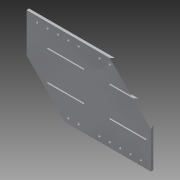
# Autodesk Inventor part: LiDAR Plate
Saved by Autodesk Inventor 2016 (Build 200138000, 138)
## iProperties
Created: 2016-04-02
Part Number: LiDAR Plate
Material: Aluminum 6061
Document SubType Name: Modeling
Designer: hwasserb
Density: 2.71 g/cm^3
Appearance: Aluminum - Flat
Author: hwasserb
Autodesk Inventor part; units mm, degrees
ref_plane "YZ Plane" through (0, 0, 0) normal (1, 0, 0) x (0, 1, 0)
ref_plane "XZ Plane" through (0, 0, 0) normal (0, 1, 0) x (-1, 0, 0)
ref_plane "XY Plane" through (0, 0, 0) normal (0, 0, 1) x (1, 0, 0)
sketch "Sketch1" plane through (0, 0, 0) normal (0, 1, 0) x (-1, 0, 0)
  line L0 (0, 0) -> (-304.8, 0)
  line L1 (-304.8, 0) -> (-304.8, 190.5)
  line L2 (-304.8, 190.5) -> (0, 190.5)
  line L3 (0, 190.5) -> (0, 0)
  dimension "d0" = 304.8
  dimension "d1" = 190.5
  constraints: 8 end point, 2 parallel, 1 horizontal, 1 perpendicular
  measures "d0" distance of L0.start L0.end
  measures "d1" distance of L2.end L0.start
extrude "Extrusion1" add sketch "Sketch1" along normal blind 6.35
sketch "Sketch2" plane through (0, 6.35, 0) normal (0, 1, 0) x (1, 0, 0)
  line L0 (304.8, 0) -> (0, 0) projected
  line L1 (0, 0) -> (0, -190.5) projected
  line L2 (0, -190.5) -> (304.8, -190.5) projected
  line L3 (304.8, -190.5) -> (304.8, 0) projected
  point P0 (25.4, -12.7)
  point P1 (50.8, -12.7)
  point P2 (76.2, -12.7)
  point P3 (101.6, -12.7)
  point P4 (127, -12.7)
  point P5 (177.8, -12.7)
  point P6 (203.2, -12.7)
  point P7 (228.6, -12.7)
  point P8 (254, -12.7)
  point P9 (279.4, -12.7)
  point P10 (25.4, -177.8)
  point P11 (50.8, -177.8)
  point P12 (76.2, -177.8)
  point P13 (101.6, -177.8)
  point P14 (127, -177.8)
  point P15 (177.8, -177.8)
  point P16 (203.2, -177.8)
  point P17 (228.6, -177.8)
  point P18 (254, -177.8)
  point P19 (279.4, -177.8)
  dimension "d4" = 25.4
  dimension "d5" = 25.4
  dimension "d6" = 25.4
  dimension "d7" = 25.4
  dimension "d8" = 25.4
  dimension "d9" = 25.4
  dimension "d10" = 25.4
  dimension "d11" = 25.4
  dimension "d12" = 25.4
  dimension "d13" = 12.7
  dimension "d14" = 12.7
  dimension "d15" = 25.4
  constraints: 18 horizontal alignment, 10 vertical alignment
  measures "d4" distance of point (101.6, -12.7) point (127, -12.7)
  measures "d5" distance of point (76.2, -12.7) point (101.6, -12.7)
  measures "d6" distance of point (50.8, -12.7) point (76.2, -12.7)
  measures "d7" distance of point (25.4, -12.7) point (50.8, -12.7)
  measures "d8" distance of point (203.2, -12.7) point (177.8, -12.7)
  measures "d9" distance of point (228.6, -12.7) point (203.2, -12.7)
  measures "d10" distance of point (254, -12.7) point (228.6, -12.7)
  measures "d11" distance of point (279.4, -12.7) point (254, -12.7)
  measures "d12" distance from line of L1 point (25.4, -12.7)
  measures "d13" distance from line of L0 point (25.4, -12.7)
  measures "d14" distance from line of L2 point (25.4, -177.8)
  measures "d15" distance from line of L3 point (279.4, -12.7)
hole "Hole1" at (25.4, 6.35, 12.7) at (50.8, 6.35, 12.7) at (76.2, 6.35, 12.7) at (101.6, 6.35, 12.7) at (127, 6.35, 12.7) at (177.8, 6.35, 12.7) at (203.2, 6.35, 12.7) at (228.6, 6.35, 12.7) at (254, 6.35, 12.7) at (279.4, 6.35, 12.7) at (25.4, 6.35, 177.8) at (50.8, 6.35, 177.8) at (76.2, 6.35, 177.8) at (101.6, 6.35, 177.8) at (127, 6.35, 177.8) at (177.8, 6.35, 177.8) at (203.2, 6.35, 177.8) at (228.6, 6.35, 177.8) at (254, 6.35, 177.8) at (279.4, 6.35, 177.8) direction (0, -1, 0) diameter 6.35 end through all
sketch "Sketch3" plane through (0, 6.35, 0) normal (0, 1, 0) x (1, 0, 0)
  line L0 (304.8, 0) -> (0, 0) projected
  line L1 (0, 0) -> (0, -190.5) projected
  line L2 (50.8, -55.475) -> (139.7, -55.475) construction
  line L3 (50.8, -56.975) -> (139.7, -56.975)
  line L4 (139.7, -53.975) -> (50.8, -53.975)
  arc A0 (50.8, -53.975) -> (50.8, -56.975) centre (50.8, -55.475) ccw
  arc A1 (139.7, -56.975) -> (139.7, -53.975) centre (139.7, -55.475) ccw
  line L5 (203.2, -128.4746) -> (292.1, -128.4746) construction
  line L6 (203.2, -129.9746) -> (292.1, -129.9746)
  line L7 (292.1, -126.9746) -> (203.2, -126.9746)
  arc A2 (203.2, -126.9746) -> (203.2, -129.9746) centre (203.2, -128.4746) ccw
  arc A3 (292.1, -129.9746) -> (292.1, -126.9746) centre (292.1, -128.4746) ccw
  line L8 (203.2, -55.475) -> (292.1, -55.475) construction
  line L9 (203.2, -56.975) -> (292.1, -56.975)
  line L10 (292.1, -53.975) -> (203.2, -53.975)
  arc A4 (203.2, -53.975) -> (203.2, -56.975) centre (203.2, -55.475) ccw
  arc A5 (292.1, -56.975) -> (292.1, -53.975) centre (292.1, -55.475) ccw
  line L11 (139.7, -126.9746) -> (50.8, -126.9746)
  line L12 (50.8, -129.9746) -> (139.7, -129.9746)
  arc A6 (50.8, -126.9746) -> (50.8, -129.9746) centre (50.8, -128.4746) ccw
  line L13 (50.8, -128.4746) -> (139.7, -128.4746) construction
  arc A7 (139.7, -129.9746) -> (139.7, -126.9746) centre (139.7, -128.4746) ccw
  line L14 (50.8, -128.4746) -> (0, -190.5) construction
  point P0 (95.25, -55.475)
  point P1 (247.65, -128.4746)
  point P2 (247.65, -55.475)
  point P3 (95.25, -128.4746)
  dimension "d23" = 88.9
  dimension "d24" = 3
  dimension "d26" = 3
  dimension "d28" = 3
  dimension "d30" = 3
  dimension "d32" = 152.4
  dimension "d33" = 50.8
  dimension "d36" = 72.9996
  dimension "d37" = 53.975
  constraints: 34 end point, 16 point on circle, 16 tangent, 8 centre point, 5 parallel, 4 midpoint, 3 equal length, 2 collinear, 2 vertical alignment, 1 horizontal
  measures "d23" distance of L2.start L2.end
  measures "d24" diameter of A1
  measures "d26" diameter of A3
  measures "d28" diameter of A5
  measures "d30" diameter of A7
  measures "d32" distance of L8.start L2.start
  measures "d33" distance from line of L13.start L1
  measures "d36" distance of L13.start L2.start
  measures "d37" distance between parallel lines of L0 L4
extrude "Extrusion2" cut sketch "Sketch3" along normal through all both and the other way through all
body "Solid1"
